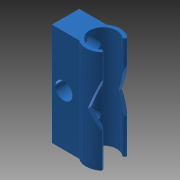
# Autodesk Inventor part: brush clip
Saved by Autodesk Inventor 2013 (Build 170138000, 138)
## iProperties
Created: 2017-01-26
Part Number: brush clip
Material: Generic
Document SubType Name: Modeling
Designer: Herman de Vries
Density: 1 g/cm^3
Author: Herman de Vries
Autodesk Inventor part; units mm, degrees
ref_plane "YZ Plane" through (0, 0, 0) normal (1, 0, 0) x (0, 1, 0)
ref_plane "XZ Plane" through (0, 0, 0) normal (0, 1, 0) x (-1, 0, 0)
ref_plane "XY Plane" through (0, 0, 0) normal (0, 0, 1) x (1, 0, 0)
sketch "Sketch1" plane through (0, 0, 0) normal (0, 0, 1) x (1, 0, 0)
  arc A0 (2.6458, 3) -> (2.6458, -3) centre (0, 0) ccw
  arc A1 (4, 3) -> (4, -3) centre (0, 0) ccw
  line L0 (-4, -3) -> (-11, -3)
  line L1 (-11, -3) -> (-11, 3)
  line L2 (-11, 3) -> (-4, 3)
  line L3 (-4, 3) -> (-4, -3)
  line L4 (2.6458, 3) -> (4, 3)
  line L5 (4, 3) -> (4, -3) construction
  line L6 (4, -3) -> (2.6458, -3)
  line L7 (2.6458, -3) -> (2.6458, 3) construction
  line L8 (-11, 3) -> (-3, 3)
  line L9 (-3, 3) -> (-3, 4)
  line L10 (-3, 4) -> (-11, 4)
  line L11 (-11, 4) -> (-11, 3)
  line L12 (-11, -3) -> (-3, -3)
  line L13 (-3, -3) -> (-3, -4)
  line L14 (-3, -4) -> (-11, -4)
  line L15 (-11, -4) -> (-11, -3)
  point P0 (2.6458, 0)
  dimension "d0" = 8
  dimension "d1" = 10
  dimension "d3" = 6
  dimension "d24" = 11
  dimension "d25" = 1
  dimension "d26" = 1
  constraints: 34 end point, 8 parallel, 8 point on circle, 4 horizontal, 4 perpendicular, 2 centre point, 2 coincident, 2 point on line, 1 horizontal alignment, 1 midpoint, 1 tangent
  measures "d0" diameter of A0
  measures "d1" diameter of A1
  measures "d3" distance of L4.end L5.end
  measures "d24" distance from line of point (0, 0) L1
  measures "d25" distance of L10.end L1.end
  measures "d26" distance of L14.end L0.end
extrude "Extrusion1" add sketch "Sketch1" along normal blind 30
sketch "Sketch2" plane through (-11, -4, 0) normal (-1, 0, 0) x (0, 0, 1)
  circle A0 centre (8, 4) radius 1.5
  circle A1 centre (26, 4) radius 1.5
  line L0 (0, 8) -> (0, 0) projected
  point P0 (0, 4)
  dimension "d6" = 3
  dimension "d9" = 3
  dimension "d10" = 18
  constraints: 2 centre point, 2 horizontal alignment, 1 midpoint
  measures "d6" diameter of A0
  measures "d9" diameter of A1
  measures "d10" distance of A1.centre A0.centre
extrude "Extrusion2" cut sketch "Sketch2" against normal blind 10
fillet "Fillet1" radius 0.5 2 edges at (4, 3, 15) (4, -3, 15)
sketch "Sketch3" plane through (-11, -4, 0) normal (0, -1, 0) x (1, 0, 0)
  circle A0 centre (3.5, 15) radius 2.5
  line L0 (0, 0) -> (0, 30)
  line L1 (0, 0) -> (7, 0)
  line L2 (19.5327, 37.0698) -> (11.5, 15)
  line L3 (19.5327, 37.0698) -> (43.0189, 37.0698) construction
  line L4 (11.5, 15) -> (19.5327, 1.0869)
  line L5 (19.5327, 1.0869) -> (19.5327, 37.0698)
  point P0 (11, 0)
  point P1 (0, 15)
  point P2 (3.5, 0)
  dimension "d14" = 5
  dimension "d17" = 110
  dimension "d18" = 130
  dimension "d19" = 8
  constraints: 12 end point, 2 horizontal alignment, 2 midpoint, 1 centre point, 1 equal length, 1 horizontal, 1 vertical, 1 vertical alignment
  measures "d14" diameter of A0
  measures "d17" angle of L2 L3
  measures "d18" angle of L4 L2
  measures "d19" distance of L2.end A0.centre
extrude "Extrusion3" cut sketch "Sketch3" along normal through all both and the other way through all
sketch "Sketch4" plane through (0, 0, 0) normal (1, 0, 0) x (0, 1, 0)
  spline S0 degree 2 poles (0, 9.5) (2.5981, 9.5) (1.299, 7.25) (0, 5) (-1.299, 7.25) (-2.5981, 9.5) (0, 9.5) knots 0 0 0 0.333333 0.333333 0.666667 0.666667 1 1 1 weights 1 0.5 1 0.5 1 0.5 1 projected
  spline S1 degree 2 poles (0, 27.5) (2.5981, 27.5) (1.299, 25.25) (0, 23) (-1.299, 25.25) (-2.5981, 27.5) (0, 27.5) knots 0 0 0 0.333333 0.333333 0.666667 0.666667 1 1 1 weights 1 0.5 1 0.5 1 0.5 1 projected
  circle A0 centre (0, 26) radius 2.5
  circle A1 centre (0, 8) radius 2.5
  point P0 (0, 0)
  dimension "d20" = 5
  dimension "d21" = 5
  constraints: 2 centre point, 2 other
  measures "d20" diameter of A0
  measures "d21" diameter of A1
extrude "Extrusion4" cut sketch "Sketch4" against normal blind 7
equation "\"d26\" = d25"
body "Solid1"
